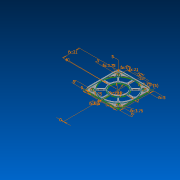
# Autodesk Inventor part: 40mm fan grill
Saved by Autodesk Inventor 2015 (Build 190159000, 159)
## iProperties
Created: 2017-03-15
Part Number: 40mm fan grill
Material: Generic
Document SubType Name: Modeling
Designer: ZigZagJoe
Density: 1 g/cm^3
Appearance: Default
Author: ZigZagJoe
Autodesk Inventor part; units mm, degrees
ref_plane "YZ Plane" through (0, 0, 0) normal (1, 0, 0) x (0, 1, 0)
ref_plane "XZ Plane" through (0, 0, 0) normal (0, 1, 0) x (-1, 0, 0)
ref_plane "XY Plane" through (0, 0, 0) normal (0, 0, 1) x (1, 0, 0)
sketch "Sketch1" plane through (0, 0, 0) normal (0, 0, 1) x (1, 0, 0)
  line L0 (-16, 21) -> (16, 21)
  line L1 (21, 16) -> (21, -16)
  line L2 (16, -21) -> (-16, -21)
  line L3 (-21, -16) -> (-21, 16)
  circle A0 centre (-16, -16) radius 1.875
  circle A1 centre (-16, 16) radius 1.875
  circle A2 centre (16, 16) radius 1.875
  circle A3 centre (16, -16) radius 1.875
  circle A4 centre (0, 0) radius 20
  arc A5 (-16, 21) -> (-21, 16) centre (-16, 16) ccw
  arc A6 (21, 16) -> (16, 21) centre (16, 16) ccw
  arc A7 (16, -21) -> (21, -16) centre (16, -16) ccw
  arc A8 (-21, -16) -> (-16, -21) centre (-16, -16) ccw
  circle A9 centre (0, 0) radius 11
  circle A10 centre (0, 0) radius 9.8
  line L4 (-0.6, -10.9836) -> (-0.6, -19.991)
  line L5 (0.6, -10.9836) -> (0.6, -19.991)
  point P0 (21, -21)
  point P1 (21, 21)
  point P2 (-21, -21)
  dimension "d0" = 42
  dimension "d1" = 42
  dimension "d2" = 3.75
  dimension "d3" = 3.75
  dimension "d4" = 3.75
  dimension "d5" = 3.75
  dimension "d6" = 40
  dimension "d7" = 32
  dimension "d8" = 32
  dimension "d9" = 5
  dimension "d11" = 5
  dimension "d12" = 5
  dimension "d13" = 5
  dimension "d14" = 5
  dimension "d15" = 5
  dimension "d16" = 21
  dimension "d17" = 21
  dimension "d18" = 5
  dimension "d19" = 5
  dimension "d20" = 22
  dimension "d21" = 19.6
  dimension "d22" = 1.2
  dimension "d23" = 0.6
  dimension "d44" = 0
  dimension "d45" = 0
  constraints: 12 end point, 12 point on circle, 11 centre point, 8 tangent, 6 point on line, 3 equal radius, 3 parallel, 2 coincident, 1 horizontal, 1 perpendicular, 1 vertical
  measures "d0" distance of point (21, -21) point (-21, -21)
  measures "d1" distance of point (21, 21) point (21, -21)
  measures "d2" diameter of A0
  measures "d3" diameter of A1
  measures "d4" diameter of A2
  measures "d5" diameter of A3
  measures "d6" diameter of A4
  measures "d7" distance of A2.centre A1.centre
  measures "d8" distance of A3.centre A0.centre
  measures "d9" distance from line of L3 A1.centre
  measures "d11" distance from line of L0 A1.centre
  measures "d12" distance from line of L0 A2.centre
  measures "d13" distance from line of L1 A2.centre
  measures "d14" distance from line of L2 A0.centre
  measures "d15" distance from line of L3 A0.centre
  measures "d16" distance from line of L3 A4.centre
  measures "d17" distance from line of L0 A4.centre
  measures "d18" distance from line of L2 A3.centre
  measures "d19" radius of A5
  measures "d20" diameter of A9
  measures "d21" diameter of A10
  measures "d22" distance between parallel lines of L5 L4
  measures "d23" distance from line of L4 A9.centre
  measures "d44" distance of point (0, 0) A4.centre
  measures "d45" distance of A4.centre point (0, 0)
extrude "Extrusion1" add sketch "Sketch1" along normal blind 1.5 contours L0 A6 L1 A7 L2 A8 L3 A5 | A9
extrude "Extrusion2" add sketch "Sketch1" along normal blind 1.5 contours L4 A9 L5 A4 picked at (0.4667, -13.9909)
fillet "Fillet1" radius 2 4 edges at (-0.6, -10.9836, 0.75) (0.6, -10.9836, 0.75) (0.6, -19.991, 0.75) (-0.6, -19.991, 0.75)
pattern_circular "Circular Pattern2" count 8 over 360 about axis through (0, 0, -10) along (0, 0, 1) of "Extrusion2", "Fillet1"
equation "\"d3\" = d2"
equation "\"d4\" = d2"
equation "\"d5\" = d2"
equation "\"d9\" = d13"
equation "\"d12\" = d11"
equation "\"d16\" = 0.5 * d0"
equation "\"d17\" = 0.5 * d0"
equation "\"d23\" = 0.5 * d22"
body "Solid1"
